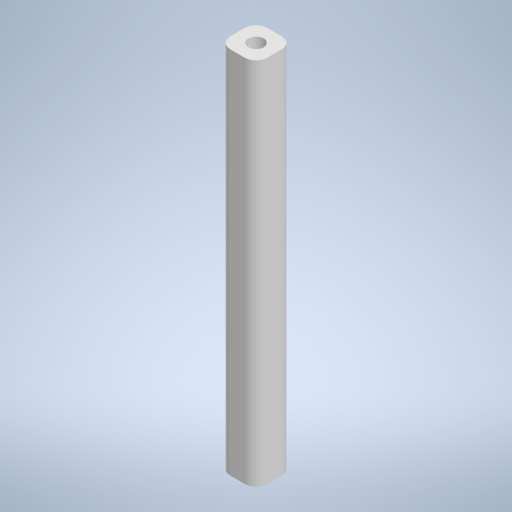
# Autodesk Inventor part: Columna
Saved by Autodesk Inventor 2024 (Build 280153000, 153)
## iProperties
Created: 2025-02-23
Part Number: Columna
Material: Genérico
Document SubType Name: Modeling
Designer: sergi
Density: 1 g/cm^3
Appearance: Valor por defecto
Author: sergi
Autodesk Inventor part; units mm, degrees
ref_plane "YZ Plane" through (0, 0, 0) normal (1, 0, 0) x (0, 1, 0)
ref_plane "XZ Plane" through (0, 0, 0) normal (0, 1, 0) x (-1, 0, 0)
ref_plane "XY Plane" through (0, 0, 0) normal (0, 0, 1) x (1, 0, 0)
sketch "Boceto1" plane through (0, 0, 0) normal (0, 1, 0) x (-1, 0, 0)
  line L0 (-2, -5) -> (2, -5)
  line L1 (5, -2) -> (5, 2)
  line L2 (2, 5) -> (-2, 5)
  line L3 (-5, 2) -> (-5, -2)
  line L4 (-5, -5) -> (5, 5) construction
  line L5 (5, -5) -> (-5, 5) construction
  arc A0 (5, 2) -> (2, 5) centre (2, 2) ccw
  arc A1 (2, -5) -> (5, -2) centre (2, -2) ccw
  arc A2 (-5, -2) -> (-2, -5) centre (-2, -2) ccw
  arc A3 (-2, 5) -> (-5, 2) centre (-2, 2) ccw
  point P0 (0, 0)
  dimension "d0" = 10
  dimension "d1" = 10
  dimension "d2" = 3
  constraints: 12 end point, 8 point on circle, 8 point on line, 8 tangent, 4 centre point, 3 equal radius, 2 midpoint, 2 parallel, 1 horizontal, 1 perpendicular
  measures "d0" distance of L5.end L4.end
  measures "d1" distance of L4.end L5.start
  measures "d2" radius of A0
extrude "Extrusión1" add sketch "Boceto1" along normal blind 100
sketch "Boceto2" plane through (0, 100, 0) normal (0, 1, 0) x (1, 0, 0)
  line L0 (2, 5) -> (-2, 5) projected
  line L1 (5, -2) -> (5, 2) projected
  point P0 (0, 0)
  point P1 (0, 0)
  dimension "d5" = 5
  dimension "d6" = 5
  measures "d5" distance from line of L0 point (0, 0)
  measures "d6" distance from line of L1 point (0, 0)
hole "Agujero1" at (0, 100, 0) direction (0, -1, 0) diameter 4.2 depth 20 tip angle 118
sketch "Boceto3" plane through (0, 0, 0) normal (0, -1, 0) x (1, 0, 0)
  line L0 (5, 2) -> (5, -2) projected
  line L1 (-2, 5) -> (2, 5) projected
  point P0 (0, 0)
  point P1 (0, 0)
  dimension "d14" = 5
  dimension "d15" = 5
  measures "d14" distance from line of L0 point (0, 0)
  measures "d15" distance from line of L1 point (0, 0)
hole "Agujero2" at (0, 0, 0) direction (0, 1, 0) diameter 4.2 depth 20 tip angle 118
